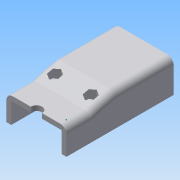
# Autodesk Inventor part: part2_bottom
Saved by Autodesk Inventor 2015 (Build 190159000, 159)
## iProperties
Created: 2015-08-21
Part Number: part2_bottom
Material: Générique
Document SubType Name: Modeling
Designer: Gregwar
Density: 1 g/cm^3
Appearance: Par défaut
Author: Gregwar
Autodesk Inventor part; units mm, degrees
ref_plane "YZ Plane" through (0, 0, 0) normal (1, 0, 0) x (0, 1, 0)
ref_plane "XZ Plane" through (0, 0, 0) normal (0, 1, 0) x (-1, 0, 0)
ref_plane "XY Plane" through (0, 0, 0) normal (0, 0, 1) x (1, 0, 0)
sketch "Esquisse1" plane through (0, 0, 0) normal (0, 1, 0) x (-1, 0, 0)
  line L0 (0, 0) -> (37, 0)
  line L1 (37, 0) -> (37, -39.5)
  line L2 (37, -39.5) -> (0, -39.5)
  line L3 (0, -39.5) -> (0, 0)
  line L4 (34, -36.5) -> (34, -3)
  line L5 (34, -3) -> (3, -3)
  line L6 (3, -3) -> (3, -36.5)
  line L7 (3, -36.5) -> (34, -36.5)
  line L8 (3, -19.75) -> (0, -19.75)
  line L9 (34, -19.75) -> (37, -19.75)
  dimension "d0" = 3
  dimension "d1" = 31
  dimension "d38" = 16.75
  constraints: 20 end point, 4 midpoint, 4 parallel, 2 perpendicular, 1 horizontal, 3 other
  measures "d0" distance between parallel lines of L7 L2
  measures "d1" distance of L4.end L5.end
  measures "d38" distance between parallel lines of L8 L5
extrude "Extrusion1" add sketch "Esquisse1" along normal blind 66 contours L0 L1 L9 L4 L5 L6 L8 L3
sketch "Esquisse2" plane through (-37, 0, 0) normal (0, 0, 1) x (1, 0, 0)
  line L0 (7.5, 22.5) -> (29.5, 22.5) construction
  circle A0 centre (7.5, 22.5) radius 1.65
  circle A1 centre (29.5, 22.5) radius 1.65
  line L1 (34, 0) -> (3, 0) construction
  line L2 (18.5, 0) -> (18.5, 22.5) construction
  point P0 (37, 0)
  dimension "d5" = 3.3
  dimension "d6" = 22.5
  dimension "d7" = 22
  constraints: 4 end point, 2 centre point, 2 coincident, 2 midpoint, 1 equal radius, 1 perpendicular, 1 vertical
  measures "d5" diameter of A1
  measures "d6" distance of L2.start L2.end
  measures "d7" distance of A0.centre A1.centre
extrude "Extrusion2" cut sketch "Esquisse2" against normal through all
sketch "Esquisse3" plane through (-33, 0, 0) normal (0, 0, 1) x (1, 0, 0)
  line L0 (-4, 66) -> (33, 66) construction
  line L1 (-4, 0) -> (33, 0) construction
  circle A0 centre (3.5, 22.5) radius 1.65 construction
  circle A1 centre (25.5, 22.5) radius 1.65 construction
  circle A2 centre (3.5, 22.5) radius 1.65 construction
  circle A3 centre (3.5, 22.5) radius 3.15
  circle A4 centre (25.5, 22.5) radius 3.15
  line L2 (33, 0) -> (33, 66) projected
  line L3 (-4, 0) -> (-4, 66) projected
  dimension "d11" = 6.3
  constraints: 2 centre point, 2 coincident, 1 equal radius
  measures "d11" diameter of A4
extrude "Extrusion3" cut sketch "Esquisse3" against normal blind 1
sketch "Esquisse7" plane through (0, 0, 0) normal (1, 0, 0) x (0, 0, -1)
  line L0 (3, 0) -> (3, 66) construction
  line L1 (0, 0) -> (19.75, 0) construction
  line L2 (19.75, 0) -> (19.75, 66) construction
  line L3 (0, 66) -> (19.75, 66) construction
  line L4 (0, 0) -> (0, 66) construction
  line L5 (19.75, 0) -> (3, 0) projected
  line L6 (4, 0) -> (4, 15)
  line L7 (4, 15) -> (2, 20) construction
  line L8 (0, 0) -> (0, 66) projected
  line L9 (2, 20) -> (0, 30) construction
  spline S0 degree 2 poles (4, 15) (2, 20) (0, 30) knots 1 1 1 2 2 2
  line L10 (0, 30) -> (0, 0)
  line L11 (0, 0) -> (4, 0)
  line L12 (0, 0) -> (19.75, 0) projected
  dimension "d39" = 15
  dimension "d41" = 30
  dimension "d42" = 4
  dimension "d43" = 2
  dimension "d44" = 20
  constraints: 6 end point, 2 collinear, 2 point on line, 1 perpendicular, 3 other
  measures "d39" distance of L6.start L6.end
  measures "d41" distance of L8.start L9.end
  measures "d42" distance between parallel lines of L10 L6
  measures "d43" distance from line of L6 L7.end
  measures "d44" distance from line of L1 L7.end
extrude "Extrusion7" cut sketch "Esquisse7" against normal through all
sketch "Esquisse8" plane through (0, 0, -19.75) normal (1, 0, 0) x (0, 0, -1)
  spline S0 degree 2 poles (-19.75, 30) (-17.75, 20) (-15.75, 15) knots 0 0 0 1 1 1 projected
  line L0 (-15.75, 15) -> (-15.75, 0) projected
  line L1 (-35.7394, 11.5677) -> (-35.7394, 0)
  line L2 (-19.75, 30) -> (-19.75, 66) projected
  line L3 (-19.75, 33) -> (-12.75, 15)
  line L4 (-12.75, 15) -> (-12.75, 0)
  line L5 (-12.75, 0) -> (-15.75, 0)
  line L6 (-15.75, 0) -> (-15.75, 15) projected
  line L7 (-19.75, 33) -> (-19.75, 30)
  line L8 (-15.75, 15) -> (-12.75, 15) construction
  point P0 (-19.75, 0)
  point P1 (-34.3097, 7.5761)
  dimension "d47" = 3
  dimension "d48" = 3
  constraints: 12 end point, 2 parallel, 2 perpendicular, 1 collinear, 1 point on line, 4 other
  measures "d47" distance between parallel lines of L0 L4
  measures "d48" distance of L2.start L3.start
extrude "Extrusion8" add sketch "Esquisse8" against normal blind 35
sketch "Esquisse9" plane through (-33, 0, -4) normal (0, 0, 1) x (1, 0, 0)
  line L0 (33, 0) -> (-4, 0) projected
  circle A0 centre (14.5, 0) radius 3.5
  point P0 (29, 0)
  point P1 (0, 0)
  dimension "d53" = 7
  constraints: 1 centre point, 1 midpoint
  measures "d53" diameter of A0
extrude "Extrusion9" cut sketch "Esquisse9" against normal through all
sketch "Esquisse10" plane through (-37, 66, 0) normal (0, 0, 1) x (1, 0, 0)
  point P0 (37, -66)
sketch "Esquisse12" plane through (0, 0, -19.75) normal (1, 0, 0) x (0, 0, -1)
  spline S0 degree 2 poles (-19.75, 30) (-17.75, 20) (-15.75, 15) knots 0 0 0 1 1 1 projected
  line L0 (-19.75, 30) -> (-12.75, 26)
  line L1 (-12.75, 26) -> (-12.75, 15)
  line L2 (-12.75, 15) -> (-15.75, 15)
  line L3 (-15.75, 15) -> (-15.75, 0) projected
  point P0 (-19.75, 0)
  dimension "d61" = 3
  dimension "d62" = 4
  constraints: 6 end point, 1 parallel, 1 perpendicular, 1 other
  measures "d61" distance between parallel lines of L3 L1
  measures "d62" vertical distance of L0.start L0.end
extrude "Extrusion11" add sketch "Esquisse12" against normal blind 35
sketch "Esquisse11" plane through (-37, 66, 0) normal (0, 0, 1) x (1, 0, 0)
  line L0 (0, -66) -> (37, -66) construction
  line L1 (37, -66) -> (22, -66) construction
  line L2 (18.5, -66) -> (18.5, 0) construction
  line L3 (34, 0) -> (3, 0) construction
  line L4 (7.5, -43.5) -> (29.5, -43.5) construction
  line L5 (29.5, -47.1373) -> (26.35, -45.3187)
  line L6 (26.35, -45.3187) -> (26.35, -41.6813)
  line L7 (26.35, -41.6813) -> (29.5, -39.8627)
  line L8 (29.5, -39.8627) -> (32.65, -41.6813)
  line L9 (32.65, -41.6813) -> (32.65, -45.3187)
  line L10 (32.65, -45.3187) -> (29.5, -47.1373)
  line L11 (10.65, -45.3187) -> (7.5, -47.1373)
  line L12 (7.5, -47.1373) -> (4.35, -45.3187)
  line L13 (4.35, -45.3187) -> (4.35, -41.6813)
  line L14 (4.35, -41.6813) -> (7.5, -39.8627)
  line L15 (7.5, -39.8627) -> (10.65, -41.6813)
  line L16 (10.65, -41.6813) -> (10.65, -45.3187)
  line L17 (0, -66) -> (0, 0) projected
  point P0 (18.5, -43.5)
  dimension "d56" = 22.5
  dimension "d57" = 22
  dimension "d69" = 6.3
  constraints: 30 end point, 3 midpoint, 3 parallel, 2 coincident, 1 collinear, 1 perpendicular, 1 point on line, 26 other
  measures "d56" distance between parallel lines of L0 L4
  measures "d57" distance of L4.end L4.start
  measures "d69" distance between parallel lines of L13 L16
extrude "Extrusion10" cut sketch "Esquisse11" against normal blind 6.3
sketch "Esquisse13" plane through (0, 0, -4) normal (0, 0, 1) x (1, 0, 0)
  circle A0 centre (-29.5, 22.5) radius 3.5 projected
  circle A1 centre (-7.5, 22.5) radius 3.5 projected
  circle A2 centre (-29.5, 22.5) radius 1.65
  circle A3 centre (-7.5, 22.5) radius 1.65
  point P0 (0, 0)
  dimension "d65" = 3.3
  constraints: 2 centre point, 2 coincident, 1 equal radius
  measures "d65" diameter of A2
extrude "Extrusion12" cut sketch "Esquisse13" against normal through all contours A2 | A3
fillet "Congé7" radius 4 6 edges at (0, 48, 0) (0, 21.25, -2) (0, 7.5, -4) (-37, 48, 0) (-37, 22.4118, -1.6978) (-37, 7.5, -4)
